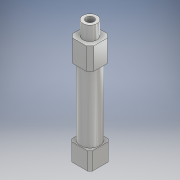
# Autodesk Inventor part: air_cylinder_15_part1_sa
Saved by Autodesk Inventor 2018 (Build 220112000, 112)
## iProperties
Created: 2018-01-19
Part Number: air_cylinder_15_part1_sa
Material: アルミニウム 6061-AHC
Document SubType Name: Modeling
Designer: shun
Density: 2.7 g/cm^3
Appearance: アルミニウム - ダーク
Author: shun
Autodesk Inventor part; units mm, degrees
ref_plane "YZ Plane" through (0, 0, 0) normal (1, 0, 0) x (0, 1, 0)
ref_plane "XZ Plane" through (0, 0, 0) normal (0, 1, 0) x (-1, 0, 0)
ref_plane "XY Plane" through (0, 0, 0) normal (0, 0, 1) x (1, 0, 0)
sketch "スケッチ1" plane through (0, 0, 0) normal (0, 0, 1) x (1, 0, 0)
  circle A0 centre (0, 0) radius 4
  dimension "d0" = 8
  constraints: 1 centre point, 1 coincident
  measures "d0" diameter of A0
extrude "押し出し1" add sketch "スケッチ1" along normal blind 8
sketch "スケッチ2" plane through (0, 0, 0) normal (0, 0, 1) x (1, 0, 0)
  line L0 (-6, -6) -> (6, -6)
  line L1 (6, -6) -> (6, 6)
  line L2 (6, 6) -> (-6, 6)
  line L3 (-6, 6) -> (-6, -6)
  line L4 (-6, -6) -> (6, 6) construction
  line L5 (6, -6) -> (-6, 6) construction
  point P0 (0, 0)
  dimension "d3" = 12
  dimension "d4" = 12
  constraints: 12 end point, 2 midpoint, 2 parallel, 1 horizontal, 1 perpendicular
  measures "d3" distance of L2.end L1.end
  measures "d4" distance of L1.end L0.end
extrude "押し出し2" add sketch "スケッチ2" against normal blind 12.5
chamfer "面取り1" distance 2.1 angle 45 1 edges at (6, 6, -6.25)
chamfer "面取り2" distance 2.1 angle 45 1 edges at (-6, 6, -6.25)
chamfer "面取り3" distance 2.1 angle 45 1 edges at (-6, -6, -6.25)
chamfer "面取り4" distance 2.1 angle 45 1 edges at (6, -6, -6.25)
sketch "スケッチ3" plane through (0, 0, -12.5) normal (0, 0, -1) x (-1, 0, 0)
  circle A0 centre (0, 0) radius 5.5
  dimension "d19" = 11
  constraints: 1 centre point, 1 coincident
  measures "d19" diameter of A0
extrude "押し出し3" add sketch "スケッチ3" along normal blind 38.75
sketch "スケッチ4" plane through (0, 0, -51.25) normal (0, 0, -1) x (-1, 0, 0)
  line L0 (5.875, 5.875) -> (-5.875, 5.875)
  line L1 (-5.875, 5.875) -> (-5.875, -5.875)
  line L2 (-5.875, -5.875) -> (5.875, -5.875)
  line L3 (5.875, -5.875) -> (5.875, 5.875)
  line L4 (5.875, 5.875) -> (-5.875, -5.875) construction
  line L5 (-5.875, 5.875) -> (5.875, -5.875) construction
  point P0 (0, 0)
  dimension "d22" = 11.75
  dimension "d23" = 11.75
  constraints: 12 end point, 2 midpoint, 2 parallel, 1 horizontal, 1 perpendicular
  measures "d22" distance of L2.end L1.end
  measures "d23" distance of L1.end L0.end
extrude "押し出し4" add sketch "スケッチ4" along normal blind 10
chamfer "面取り5" distance 1.4 angle 45 1 edges at (-5.875, -5.875, -56.25)
chamfer "面取り6" distance 1.4 angle 45 1 edges at (-5.875, 5.875, -56.25)
chamfer "面取り7" distance 1.4 angle 45 1 edges at (5.875, -5.875, -56.25)
chamfer "面取り8" distance 1.4 angle 45 1 edges at (5.875, 5.875, -56.25)
sketch "スケッチ5" plane through (3.9, 6, 0) normal (0, 1, 0) x (1, 0, 0)
  circle A0 centre (-3.9, 8) radius 2
  point P0 (-3.9, 0)
  dimension "d38" = 4
  dimension "d39" = 8
  constraints: 1 centre point
  measures "d38" diameter of A0
  measures "d39" distance of point (-3.9, 0) A0.centre
extrude "押し出し5" cut sketch "スケッチ5" against normal blind 10
sketch "スケッチ6" plane through (-4.475, 5.875, -51.25) normal (0, 1, 0) x (1, 0, 0)
  circle A0 centre (4.475, 5) radius 2
  line L0 (0, 0) -> (8.95, 0) projected
  point P0 (4.475, -51.25)
  dimension "d42" = 4
  dimension "d43" = 5
  constraints: 1 centre point
  measures "d42" diameter of A0
  measures "d43" distance from line of L0 A0.centre
extrude "押し出し6" cut sketch "スケッチ6" against normal blind 10
sketch "スケッチ7" plane through (0, 0, 8) normal (0, 0, 1) x (1, 0, 0)
  circle A0 centre (0, 0) radius 2.25
  dimension "d46" = 4.5
  constraints: 1 centre point, 1 coincident
  measures "d46" diameter of A0
extrude "押し出し7" cut sketch "スケッチ7" against normal blind 40
